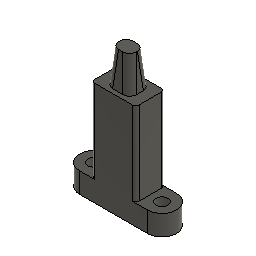
4056-USB-C-to-micro-B (Autodesk Fusion 360 design; units mm, degrees)
Autodesk Fusion 360 part; units mm, degrees
sketch "Sketch1" plane through (0, 0, 0) normal (0, 0, 1) x (1, 0, 0)
  line L0 (-10, 0) -> (10, 0) construction
  circle A0 centre (-10, 0) radius 1.75
  circle A1 centre (10, 0) radius 1.75
  line L1 (-10, 4.25) -> (10, 4.25)
  line L2 (10, 4.25) -> (10, -4.25)
  line L3 (10, -4.25) -> (-10, -4.25)
  line L4 (-10, -4.25) -> (-10, 4.25)
  line L5 (0, 4.25) -> (0, 0) construction
  arc A2 (-10, 4.25) -> (-10, -4.25) centre (-10, 0) ccw
  arc A3 (10, -4.25) -> (10, 4.25) centre (10, 0) ccw
  dimension "d1" = 20
  dimension "d2" = 3.5
  dimension "d4" = 8.5
  constraint horizontal L0
  constraint midpoint L5.end L0
  constraint coincident L0.start A0.centre
  constraint coincident L0.end A1.centre
  constraint equal A0 A1
  constraint horizontal L1
  constraint vertical L2
  constraint horizontal L3
  constraint vertical L4
  constraint midpoint L1 L5.start
  constraint coincident L5.end origin
  constraint vertical L5
  constraint midpoint L0.start L4
  constraint tangent L1 A2
  constraint symmetric L1.start L5 L1.end
  constraint symmetric L3.end L5 L2.end
  constraint symmetric L5 A2 A3
  measures "d1" distance of L0.start L0.end
  measures "d2" diameter of A0
  measures "d4" distance of L1.start L3.end
extrude "Extrude1" add sketch "Sketch1" along normal blind 6 contours A0 A1 L1 L2 L3 L4 | A0 L4 A2 | A1 L2 A3 makes body 1
sketch "Sketch2" plane through (0, 0, 0) normal (0, 0, 1) x (1, 0, 0)
  line L0 (-6.5, 4.25) -> (6.5, 4.25)
  line L1 (6.5, 4.25) -> (6.5, -4.25)
  line L2 (6.5, -4.25) -> (-6.5, -4.25)
  line L3 (-6.5, -4.25) -> (-6.5, 4.25)
  line L4 (0, 4.25) -> (0, 0) construction
  line L5 (0, 0) -> (-6.5, 0) construction
  dimension "d7" = 13
  dimension "d8" = 8.5
  constraint horizontal L0
  constraint vertical L1
  constraint horizontal L2
  constraint vertical L3
  constraint midpoint L0 L4.start
  constraint perpendicular L0 L4
  constraint midpoint L3 L5.end
  constraint perpendicular L3 L5
  constraint coincident L4.end L5.start
  measures "d7" distance of L0.start L0.end
  measures "d8" distance of L0.start L2.end
extrude "Extrude2" add sketch "Sketch2" along normal blind 40.5 bodies 1
sketch "Sketch3" plane through (0, 0, 0) normal (0, 0, 1) x (1, 0, 0)
  line L0 (3, -2) -> (-3, -2)
  line L1 (-3, -2) -> (-3, 2) construction
  line L2 (-3, 2) -> (3, 2)
  line L3 (3, 2) -> (3, -2) construction
  arc A0 (-3, 2) -> (-3, -2) centre (-3, 0) ccw
  arc A1 (3, -2) -> (3, 2) centre (3, 0) ccw
  line L4 (0, -2) -> (0, 0) construction
  line L5 (0, 0) -> (3, 0) construction
  dimension "d13" = 6
  dimension "d14" = 4
  constraint horizontal L0
  constraint vertical L1
  constraint horizontal L2
  constraint vertical L3
  constraint midpoint L0 L4.start
  constraint perpendicular L0 L4
  constraint coincident A1.centre L5.end
  constraint perpendicular L3 L5
  constraint coincident L4.end L5.start
  measures "d13" distance of L0.start L0.end
  measures "d14" distance of L0.start L2.end
extrude "Extrude3" add sketch "Sketch3" against normal blind 1 thin wall 1 centred separate body open curves L0 A1 L2 A0 makes body 2
extrude "Extrude4" cut sketch "Sketch3" along normal blind 3 bodies 1
sketch "Sketch4" plane through (0, 0, 0) normal (0, 1, 0) x (1, 0, 0)
  line L0 (6.5, -40.5) -> (-6.5, -40.5)
  line L1 (-6.5, -6) -> (-6.5, -40.5)
  line L2 (6.5, -6) -> (6.5, -40.5)
  line L3 (-3.5, -40.5) -> (-3.5, -30.5)
  line L4 (-3.5, -30.5) -> (-6.5, -30.5)
  line L5 (0, -40.5) -> (0, -29) construction
  line L6 (3.5, -40.5) -> (3.5, -30.5)
  line L7 (3.5, -30.5) -> (6.5, -30.5)
  line L8 (-3.5, -30.5) -> (3.5, -30.5)
  dimension "d20" = 3
  dimension "d21" = 10
  constraint coincident L0 L3.start
  constraint perpendicular L0 L3
  constraint coincident L1 L4.end
  constraint perpendicular L1 L4
  constraint midpoint L0 L5.start
  constraint perpendicular L0 L5
  constraint symmetric L3.start L5 L6.start
  constraint symmetric L3.end L5 L6.end
  constraint symmetric L4.end L5 L7.end
  measures "d20" distance of L1 L3
  measures "d21" distance of L3.start L3.end
extrude "Extrude6" cut sketch "Sketch4" along normal mid plane 12 bodies 1
extrude "Extrude7" add sketch "Sketch4" along normal mid plane 6 contours L0 L3 L6 L8 bodies 1
draft "Draft1" angle 5 neutral plane through (3.5, 0, 30.5) pull (0, 0, 1) 4 faces at (1.1667, -3, 37.1667) (3.5, 1, 33.8333) (1.1667, 3, 37.1667) (-3.5, -1, 37.1667) on bodies 1
fillet "Fillet3" radius 1 4 edges at (6.5, 4.25, 18.25) (-6.5, 4.25, 18.25) (-6.5, -4.25, 18.25) (6.5, -4.25, 18.25) on bodies 1
fillet "Fillet4" radius 2 4 edges at (-3.0626, -2.5626, 35.5) (-3.0626, 2.5626, 35.5) (3.0626, -2.5626, 35.5) (3.0626, 2.5626, 35.5) on bodies 1
